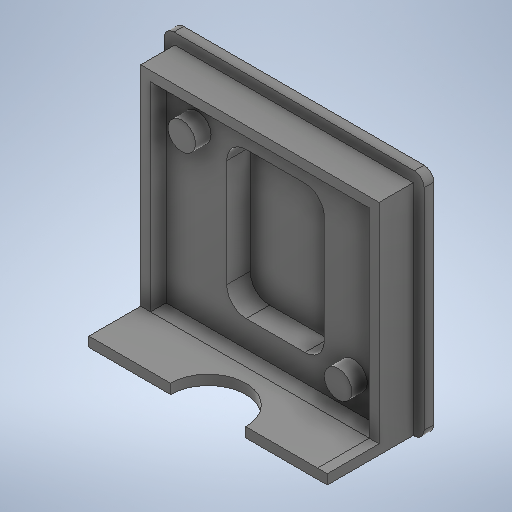
# Autodesk Inventor part: buttom cover
Saved by Autodesk Inventor 2025.4 (Build 294407000, 407)
## iProperties
Created: 2025-07-29
Part Number: buttom cover
Material: Generic
Document SubType Name: Modeling
Designer: Yuhsuan Chen
Density: 1 g/cm^3
Appearance: Default
Author: Yuhsuan Chen
Autodesk Inventor part; units mm, degrees
ref_plane "YZ Plane" through (0, 0, 0) normal (1, 0, 0) x (0, 1, 0)
ref_plane "XZ Plane" through (0, 0, 0) normal (0, 1, 0) x (-1, 0, 0)
ref_plane "XY Plane" through (0, 0, 0) normal (0, 0, 1) x (1, 0, 0)
sketch "Sketch1" plane through (0, 0, 0) normal (0, 0, 1) x (1, 0, 0)
  circle A0 centre (8, -7) radius 1.6 projected
  circle A1 centre (-8, 7) radius 1.6 projected
  circle A2 centre (-2.5, 4.7) radius 0.8 projected
  circle A3 centre (2.5001, 4.7) radius 0.8 projected
  line L0 (-11, 10) -> (-11, -10) projected
  line L1 (-11, -10) -> (11, -10) projected
  line L2 (11, -10) -> (11, 10) projected
  line L3 (11, 10) -> (-11, 10) projected
  line L4 (-11.2, -10.2) -> (-11.2, 10.2)
  line L5 (-11.2, 10.2) -> (11.2, 10.2)
  line L6 (11.2, 10.2) -> (11.2, -10.2)
  line L7 (11.2, -10.2) -> (-11.2, -10.2)
  circle A4 centre (-8, 7) radius 1.4
  circle A5 centre (8, -7) radius 1.4
  line L8 (-12.2, 11.2) -> (-12.2, -11.2)
  line L9 (-12.2, -11.2) -> (12.2, -11.2)
  line L10 (12.2, -11.2) -> (12.2, 11.2)
  line L11 (12.2, 11.2) -> (-12.2, 11.2)
  circle A6 centre (2.54, -5.9) radius 0.4 projected
  circle A7 centre (-2.54, -5.9) radius 0.4 projected
  circle A8 centre (0, -5.9) radius 0.4 projected
  circle A9 centre (3.5, -7.425) radius 0.5 projected
  circle A10 centre (-3.5, -7.425) radius 0.5 projected
  circle A11 centre (0.6, -3.225) radius 0.3 projected
  circle A12 centre (0.6, -4.425) radius 0.3 projected
  circle A13 centre (-0.6, -3.225) radius 0.3 projected
  circle A14 centre (-0.6, -4.425) radius 0.3 projected
  point P0 (0, 0)
  dimension "d6" = 15
  dimension "d7" = 10
  dimension "d0" = 0.2
  dimension "d1" = 0.2
  dimension "d2" = 0.2
  dimension "d3" = 1
  constraints: 16 end point, 2 centre point, 6 other
  measures "d0" distance between parallel lines of L0 L4
  measures "d1" radial gap between concentric circles of A1 A4
  measures "d2" radial gap between concentric circles of A0 A5
  measures "d3" distance between parallel lines of L4 L8
extrude "Extrusion1" add sketch "Sketch1" against normal blind 4 contours A4 | A5 | L11 L10 L9 L8
sketch "Sketch2" plane through (0, 0, -4) normal (0, 0, -1) x (-1, 0, 0)
  line L0 (-12.2, -11.2) -> (12.2, -11.2) projected
  line L1 (12.2, -11.2) -> (12.2, 11.2) projected
  line L2 (12.2, 11.2) -> (-12.2, 11.2) projected
  line L3 (-12.2, 11.2) -> (-12.2, -11.2) projected
  line L4 (11.2, 10.2) -> (11.2, -10.2) projected
  line L5 (11.2, -10.2) -> (-11.2, -10.2) projected
  line L6 (-11.2, -10.2) -> (-11.2, 10.2) projected
  line L7 (-11.2, 10.2) -> (11.2, 10.2) projected
  line L8 (5, -7.5) -> (-5, -7.5)
  line L9 (-5, -7.5) -> (-5, 7.5)
  line L10 (-5, 7.5) -> (5, 7.5)
  line L11 (5, 7.5) -> (5, -7.5)
  point P0 (0, 0)
  point P1 (-5, 0)
  point P2 (0, -7.5)
  point P3 (0, -11.2)
  dimension "d6" = 15
  dimension "d7" = 10
  constraints: 8 end point, 3 midpoint, 2 parallel, 1 horizontal, 1 horizontal alignment, 1 perpendicular, 1 vertical alignment
  measures "d6" distance of L8.end L9.end
  measures "d7" distance of L8.start L8.end
extrude "Extrusion2" add sketch "Sketch2" against normal blind 0.5 contours L4 L5 L6 L7
sketch "Sketch3" plane through (0, 0, -4) normal (0, 0, -1) x (-1, 0, 0)
  line L0 (5, -7.5) -> (-5, -7.5) projected
  line L1 (-5, -7.5) -> (-5, 7.5) projected
  line L2 (-5, 7.5) -> (5, 7.5) projected
  line L3 (5, 7.5) -> (5, -7.5) projected
  line L4 (-12.2, -11.2) -> (12.2, -11.2) projected
  line L5 (12.2, -11.2) -> (12.2, 11.2) projected
  line L6 (12.2, 11.2) -> (-12.2, 11.2) projected
  line L7 (-12.2, 11.2) -> (-12.2, -11.2) projected
  point P0 (0, 0)
extrude "Extrusion3" add sketch "Sketch3" along normal blind 0.5 contours L0 L1 L2 L3 | L7 L6 L5 L4
sketch "Sketch4" plane through (0, 0, 0) normal (0, 0, 1) x (1, 0, 0)
  line L0 (-12.2, -11.2) -> (12.2, -11.2) projected
  line L1 (12.2, -11.2) -> (12.2, 11.2) projected
  line L2 (12.2, 11.2) -> (-12.2, 11.2) projected
  line L3 (-12.2, 11.2) -> (-12.2, -11.2) projected
  line L4 (-11.2, -10.2) -> (-11.2, 10.2) projected
  line L5 (-11.2, 10.2) -> (11.2, 10.2) projected
  line L6 (11.2, 10.2) -> (11.2, -10.2) projected
  line L7 (11.2, -10.2) -> (-11.2, -10.2) projected
  line L8 (-11.2, -10.2) -> (-12.2, -10.2)
  line L9 (11.2, -10.2) -> (-11.2, -10.2) projected
  line L10 (11.2, -10.2) -> (12.2, -10.2)
  point P0 (0, 0)
  constraints: 4 end point, 3 point on line, 1 perpendicular
extrude "Extrusion4" add sketch "Sketch4" along normal blind 5.3 contours L3 L8 L7 L10 L1 L0
sketch "Sketch5" plane through (-12.2, -11.2, -4.5) normal (0, -1, 0) x (1, 0, 0)
  line L0 (23.4, 9.8) -> (0, 9.8) projected
  circle A0 centre (12.2, 9.8) radius 3.85
  point P0 (12.2, 4.5)
  point P1 (8.35, 9.8)
  point P2 (16.05, 9.8)
  dimension "d14" = 7.7
  constraints: 1 centre point, 1 point on line
  measures "d14" diameter of A0
extrude "Extrusion5" cut sketch "Sketch5" against normal blind 5.3 contours A0 L0 picked at (11.471, 8.7438)
sketch "Sketch6" plane through (0, 0, -4.5) normal (0, 0, -1) x (-1, 0, 0)
  line L0 (12.2, -11.2) -> (12.2, 11.2) projected
  line L1 (12.2, 11.2) -> (-12.2, 11.2) projected
  line L2 (-12.2, 11.2) -> (-12.2, -11.2) projected
  line L3 (-12.2, -11.2) -> (12.2, -11.2) projected
  line L4 (13.3, 12.3) -> (13.3, -12.3)
  line L5 (13.3, -12.3) -> (-13.3, -12.3)
  line L6 (-13.3, -12.3) -> (-13.3, 12.3)
  line L7 (-13.3, 12.3) -> (13.3, 12.3)
  line L8 (12.2, -11.2) -> (13.3, -11.2)
  line L9 (-12.2, -11.2) -> (-13.3, -11.2)
  point P0 (0, 0)
  dimension "d17" = 1.1
  constraints: 12 end point, 2 perpendicular, 2 point on line, 3 other
  measures "d17" distance between parallel lines of L0 L4
extrude "Extrusion6" add sketch "Sketch6" against normal blind 1 contours L0 L1 L2 L9 L6 L7 L4 L8
sketch "Sketch7" plane through (0, 0, -3.5) normal (0, 0, 1) x (1, 0, 0)
  circle A0 centre (8, -7) radius 1.4 projected
  circle A1 centre (-8, 7) radius 1.4 projected
  line L0 (11.2, 10.2) -> (11.2, -10.2) projected
  line L1 (-11.2, 10.2) -> (11.2, 10.2) projected
  line L2 (-11.2, -10.2) -> (-11.2, 10.2) projected
  line L3 (11.2, -10.2) -> (-11.2, -10.2) projected
  line L4 (5, -7.5) -> (-5, -7.5) projected
  line L5 (-5, -7.5) -> (-5, 7.5) projected
  line L6 (-5, 7.5) -> (5, 7.5) projected
  line L7 (5, 7.5) -> (5, -7.5) projected
  point P0 (0, 0)
extrude "Extrusion7" add sketch "Sketch7" along normal blind 1.9
fillet "Fillet1" radius 2 4 edges at (-5, 7.5, -2.8) (5, 7.5, -2.8) (-5, -7.5, -2.8) (5, -7.5, -2.8)
fillet "Fillet2" radius 1 4 edges at (13.3, 12.3, -4) (13.3, -11.2, -4) (-13.3, -11.2, -4) (-13.3, 12.3, -4)
body "Solid1"
